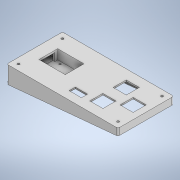
# Autodesk Inventor part: betonbase
Saved by Autodesk Inventor 2021 (Build 250183000, 183)
## iProperties
Created: 2020-07-06
Part Number: betonbase
Material: Generic
Document SubType Name: Modeling
Designer: adaml
Density: 1 g/cm^3
Appearance: Default
Author: adaml
Autodesk Inventor part; units mm, degrees
sketch "Sketch1" plane through (0, 0, 0) normal (0, 1, 0) x (-1, 0, 0)
  line L0 (-55.372, 28.575) -> (55.372, 28.575)
  line L1 (57.15, 26.797) -> (57.15, -26.797)
  line L2 (55.372, -28.575) -> (-55.372, -28.575)
  line L3 (-57.15, -26.797) -> (-57.15, 26.797)
  line L4 (-57.15, 28.575) -> (57.15, -28.575) construction
  line L5 (57.15, 28.575) -> (-57.15, -28.575) construction
  arc A0 (55.372, -28.575) -> (57.15, -26.797) centre (55.372, -26.797) ccw
  arc A1 (57.15, 26.797) -> (55.372, 28.575) centre (55.372, 26.797) ccw
  arc A2 (-57.15, -26.797) -> (-55.372, -28.575) centre (-55.372, -26.797) ccw
  arc A3 (-55.372, 28.575) -> (-57.15, 26.797) centre (-55.372, 26.797) ccw
  point P0 (0, 0)
  dimension "d0" = 114.3
  dimension "d1" = 57.15
  dimension "d2" = 1.778
  dimension "d3" = 1.778
  dimension "d4" = 1.778
  constraints: 12 end point, 8 point on circle, 8 point on line, 8 tangent, 4 centre point, 2 midpoint, 2 parallel, 1 equal radius, 1 horizontal, 1 perpendicular
  measures "d0" distance of L4.end L5.end
  measures "d1" distance of L5.start L4.end
  measures "d2" radius of A0
  measures "d3" radius of A2
  measures "d4" radius of A3
extrude "Extrusion1" add sketch "Sketch1" along normal blind 17.78
sketch "Sketch2" plane through (-55.372, 0, 28.575) normal (0, 0, 1) x (1, 0, 0)
  line L0 (112.522, 0) -> (112.522, 17.78) projected
  line L1 (112.522, 17.78) -> (112.522, 10.668)
  line L2 (0, 0) -> (-1.778, 0) projected
  line L3 (112.522, 10.668) -> (-1.778, 0)
  line L4 (-1.778, 0) -> (112.522, 0)
  line L5 (112.522, 0) -> (110.744, 0) projected
  line L6 (112.522, 10.668) -> (112.522, 0)
  point P0 (55.372, 0)
  dimension "d7" = 7.112
  constraints: 8 end point, 1 collinear, 1 point on line, 1 vertical
  measures "d7" distance of L0.end L1.end
extrude "Extrusion2" cut sketch "Sketch2" against normal blind 88.5825
sketch "Sketch4" plane through (0, 17.78, 0) normal (0, 1, 0) x (1, 0, 0)
  line L0 (-57.15, 26.797) -> (-57.15, -26.797) projected
  line L1 (-57.15, 0) -> (-51.054, 0)
  line L2 (-51.054, 0) -> (-28.702, 0)
  circle A0 centre (-28.702, 0) radius 22.352
  line L3 (-6.35, 0) -> (-1.524, 0)
  line L4 (-1.524, 0) -> (-1.524, -20.193)
  line L5 (-1.524, -20.193) -> (11.176, -20.193)
  line L6 (11.176, -20.193) -> (11.176, -13.843)
  line L7 (-1.524, -13.843) -> (11.176, -13.843)
  line L8 (11.176, -13.843) -> (11.176, 0)
  line L9 (34.544, 14.605) -> (34.544, -14.605)
  line L10 (15.494, 0) -> (34.544, 0)
  line L11 (34.544, 0) -> (15.494, 0)
  line L12 (15.494, 0) -> (15.494, 24)
  line L13 (15.494, 24) -> (34.544, 24)
  line L14 (34.544, 24) -> (34.544, 0)
  line L15 (34.544, 0) -> (15.494, 0)
  line L16 (15.494, 0) -> (15.494, -24)
  line L17 (15.494, -24) -> (34.544, -24)
  line L18 (34.544, -24) -> (34.544, 0)
  line L19 (34.544, 0) -> (53.594, 0)
  line L20 (53.594, 0) -> (53.594, -14.25)
  line L21 (53.594, -14.25) -> (34.544, -14.25)
  line L22 (34.544, -14.25) -> (34.544, 0)
  line L23 (34.544, 0) -> (53.594, 0)
  line L24 (53.594, 0) -> (53.594, 14.25)
  line L25 (53.594, 14.25) -> (34.544, 14.25)
  line L26 (34.544, 14.25) -> (34.544, 0)
  line L27 (18.019, -5) -> (32.019, -5)
  line L28 (32.019, -5) -> (32.019, -19)
  line L29 (32.019, -19) -> (18.019, -19)
  line L30 (18.019, -5) -> (32.019, -19) construction
  line L31 (32.019, -5) -> (18.019, -19) construction
  line L32 (32.019, 5) -> (18.019, 5)
  line L33 (18.019, 19) -> (32.019, 19)
  line L34 (32.019, 19) -> (32.019, 5)
  line L35 (32.019, 5) -> (18.019, 19) construction
  line L36 (18.019, 5) -> (32.019, 19) construction
  line L37 (37.069, -7) -> (51.069, -7)
  line L38 (51.069, -7) -> (51.069, 7)
  line L39 (51.069, 7) -> (37.069, 7)
  line L40 (37.069, -7) -> (51.069, 7) construction
  line L41 (51.069, -7) -> (37.069, 7) construction
  line L42 (-34.702, -6) -> (-22.702, -6)
  line L43 (-22.702, -6) -> (-22.702, 6)
  line L44 (-22.702, 6) -> (-34.702, 6)
  line L45 (-34.702, 6) -> (-34.702, -6)
  line L46 (-34.702, -6) -> (-22.702, 6) construction
  line L47 (-22.702, -6) -> (-34.702, 6) construction
  line L48 (18.269, 5.25) -> (31.769, 5.25)
  line L49 (31.769, 5.25) -> (31.769, 18.75)
  line L50 (31.769, 18.75) -> (18.269, 18.75)
  line L51 (18.269, 18.75) -> (18.269, 5.25)
  line L52 (18.269, 5.25) -> (31.769, 18.75) construction
  line L53 (31.769, 5.25) -> (18.269, 18.75) construction
  line L54 (18.269, -18.75) -> (31.769, -18.75)
  line L55 (31.769, -18.75) -> (31.769, -5.25)
  line L56 (31.769, -5.25) -> (18.269, -5.25)
  line L57 (18.269, -5.25) -> (18.269, -18.75)
  line L58 (18.269, -18.75) -> (31.769, -5.25) construction
  line L59 (31.769, -18.75) -> (18.269, -5.25) construction
  line L60 (37.319, -6.75) -> (50.819, -6.75)
  line L61 (50.819, -6.75) -> (50.819, 6.75)
  line L62 (50.819, 6.75) -> (37.319, 6.75)
  line L63 (37.319, 6.75) -> (37.319, -6.75)
  line L64 (37.319, -6.75) -> (50.819, 6.75) construction
  line L65 (50.819, -6.75) -> (37.319, 6.75) construction
  point P0 (0, 0)
  point P1 (25.019, -12)
  point P2 (25.019, 12)
  point P3 (44.069, 0)
  dimension "d15" = 6.096
  dimension "d16" = 22.352
  dimension "d17" = 4.826
  dimension "d26" = 12.7
  dimension "d52" = 19.05
  dimension "d53" = 24
  dimension "d54" = 24
  dimension "d55" = 14.25
  dimension "d56" = 14.25
  dimension "d57" = 14
  dimension "d58" = 14
  dimension "d59" = 14
  dimension "d60" = 14
  dimension "d61" = 14
  dimension "d62" = 14
  dimension "d86" = 12
  dimension "d87" = 12
  dimension "d208" = 13.5
  dimension "d209" = 13.5
  dimension "d210" = 13.5
  dimension "d211" = 13.5
  dimension "d212" = 13.5
  dimension "d213" = 13.5
  constraints: 130 end point, 19 parallel, 17 midpoint, 15 horizontal, 11 perpendicular, 2 point on circle, 2 vertical, 1 centre point, 1 coincident, 1 point on line
  measures "d15" distance of L1.start L1.end
  measures "d16" distance of L1.end L2.end
  measures "d17" distance of L3.start L3.end
  measures "d26" distance of L4.end L5.end
  measures "d52" distance of L12.end L13.end
  measures "d53" distance of L11.end L12.end
  measures "d54" distance of L16.end L15.end
  measures "d55" distance of L19.end L20.end
  measures "d56" distance of L24.end L23.end
  measures "d57" distance of L28.end L29.end
  measures "d58" distance of L27.end L28.end
  measures "d59" distance of L33.start L33.end
  measures "d60" distance of L32.end L33.start
  measures "d61" distance of L39.end L38.end
  measures "d62" distance of L38.end L37.end
  measures "d86" distance of L44.end L43.end
  measures "d87" distance of L43.end L42.end
  measures "d208" distance of L50.end L49.end
  measures "d209" distance of L49.end L48.end
  measures "d210" distance of L56.end L55.end
  measures "d211" distance of L55.end L54.end
  measures "d212" distance of L62.end L61.end
  measures "d213" distance of L61.end L60.end
shell "Shell1" thickness 2 removed faces 1 at (-18.4573, 3.6113, -9.525)
extrude "Extrusion6" cut sketch "Sketch4" against normal blind 23.8125 contours L7 L6 L5 L4 | L63 L62 L61 L19 | L19 L61 L60 L63 | L45 L44 L43 L42 | L51 L50 L49 L48 | L57 L56 L55 L54
sketch "Sketch6" plane through (-55.15, 15.78, -26.575) normal (0, -1, 0) x (1, 0, 0)
  line L0 (107.7935, 6.255) -> (70.9735, 6.255)
  line L1 (70.9735, 6.255) -> (70.9735, 46.895)
  line L2 (70.9735, 46.895) -> (107.7935, 46.895)
  line L3 (107.7935, 46.895) -> (107.7935, 6.255)
  line L4 (107.7935, 6.255) -> (70.9735, 46.895) construction
  line L5 (70.9735, 6.255) -> (107.7935, 46.895) construction
  line L6 (70.9735, 46.895) -> (51.9622, 46.895)
  line L7 (51.9622, 46.895) -> (51.9622, 6.255)
  line L8 (51.9622, 6.255) -> (70.9735, 6.255)
  line L9 (70.9735, 6.255) -> (70.9735, 46.895)
  point P0 (55.15, 26.575)
  point P1 (89.3835, 26.575)
  point P2 (70.9735, 6.255)
  dimension "d43" = 40.64
  constraints: 20 end point, 4 parallel, 2 horizontal, 2 midpoint, 2 perpendicular
  measures "d43" distance of L0.end L1.end
extrude "Extrusion7" cut sketch "Sketch6" against normal blind 0.5
ref_plane "Work Plane1" through (-57.15, 0, -26.797) normal (0.9956727, 0.0929295, 0) x (0, 0, 1)
sketch "Sketch7" plane through (-57.15, 17.78, -26.797) normal (-1, 0, 0) x (0, 0, 1)
  ellipse E0 centre (0, -17.6141) end of major axis (1.778, -17.6141) minor radius 0.1659 (-1.778, -17.6141) -> (0, -17.78) ccw projected
  line L0 (0, -17.78) -> (0, 0) projected
  line L1 (0.222, -12.7049) -> (53.372, -12.7049)
  line L2 (0, -17.78) -> (53.594, -17.78) projected
  line L3 (0.222, -12.7049) -> (0.222, -17.78)
  line L4 (26.797, -17.78) -> (26.797, -11.2738)
  line L5 (53.372, -12.7049) -> (53.372, -17.78)
  constraints: 8 end point, 2 symmetric about line, 1 perpendicular, 1 point on line, 1 vertical, 1 other
extrude "Extrusion8" cut sketch "Sketch7" against normal blind 104.775
sketch "Sketch8" plane through (-57.15, 17.78, -26.797) normal (-1, 0, 0) x (0, 0, 1)
  line L0 (0.222, -12.7049) -> (53.372, -12.7049) projected
  line L1 (6.477, -2) -> (47.117, -2) projected
  line L2 (53.372, -12.7049) -> (35.172, -12.7049)
  line L3 (44.272, -12.7049) -> (44.272, -6.5049)
  line L4 (44.272, -6.5049) -> (49.7838, -6.5049)
  line L5 (49.7838, -6.5049) -> (49.7838, -12.7049)
  line L6 (44.272, -6.5049) -> (38.7602, -6.5049)
  line L7 (38.7602, -6.5049) -> (38.7602, -12.7049)
  point P0 (26.797, -17.78)
  dimension "d91" = 18.2
  dimension "d92" = 5.5118
  dimension "d93" = 5.5118
  constraints: 12 end point, 4 point on line, 3 perpendicular, 1 midpoint, 1 vertical
  measures "d91" distance of L0.end L2.end
  measures "d92" distance of L3.end L4.end
  measures "d93" distance of L3.end L6.end
extrude "Extrusion9" cut sketch "Sketch8" against normal blind 25.4
sketch "Sketch9" plane through (-55.15, 15.78, 26.575) normal (1, 0, 0) x (0, 0, -1)
  line L0 (53.15, -10.7049) -> (0, -10.7049) projected
  line L1 (15.475, -3.5049) -> (17.475, -3.5049)
  line L2 (32.075, -4.5049) -> (32.075, -10.7049) projected
  line L3 (32.075, -7.5049) -> (32.075, -6.5049)
  line L4 (21.075, -10.7049) -> (21.075, -4.5049) projected
  line L5 (21.075, -7.5049) -> (21.075, -6.5049)
  line L6 (0, -15.78) -> (0, -5.2987) projected
  line L7 (0, -7.5049) -> (18.2, -7.5049)
  line L8 (0, -7.5049) -> (18.2, -7.5049) construction
  line L9 (18.2, -6.5049) -> (0, -6.5049)
  line L10 (18.2, -5.5049) -> (0, -5.5049)
  line L11 (14.6118, -4.5049) -> (14.6118, -10.7049) projected
  line L12 (14.6118, -8.5049) -> (14.6118, -4.5049)
  line L13 (3.5882, -10.7049) -> (3.5882, -4.5049) projected
  line L14 (3.5882, -8.5049) -> (3.5882, -4.5049)
  line L15 (18.2, -7.5049) -> (18.2, -5.5049)
  line L16 (0, -7.5049) -> (0, -5.5049)
  line L17 (18.2, -4.5049) -> (0, -4.5049)
  line L18 (18.2, -3.5049) -> (0, -3.5049)
  line L19 (18.2, -5.5049) -> (18.2, -3.5049)
  line L20 (18.2, -7.5049) -> (20.2, -7.5049)
  line L21 (20.2, -7.5049) -> (20.2, -3.5049)
  line L22 (20.2, -3.5049) -> (18.2, -3.5049)
  line L23 (0, -3.5049) -> (0, -7.5049)
  line L24 (20.2, -3.5049) -> (20.2, 0)
  line L25 (53.15, 0) -> (0, 0) projected
  line L26 (18.2, 0) -> (18.2, -3.5049)
  line L27 (20.2, 0) -> (18.2, 0)
  point P0 (26.575, -15.78)
  point P1 (3.5882, -7.5049)
  point P2 (3.5882, -6.5049)
  point P3 (14.6118, -6.5049)
  point P4 (14.6118, -7.5049)
  point P5 (17.475, -3.5049)
  point P6 (15.475, -3.5049)
  dimension "d94" = 18.2
  dimension "d95" = 0
  dimension "d96" = 2
  constraints: 42 end point, 13 point on line, 6 collinear, 3 horizontal, 3 perpendicular, 3 vertical, 2 parallel
  measures "d94" distance of L7.start L7.end
  measures "d95" distance between parallel lines of L7 L8
  measures "d96" distance of L8.end L20.end
extrude "Extrusion10" add sketch "Sketch9" along normal blind 2 contours L11 L9 L15 L7 | L6 L9 L13 L7 | L15 L19 L22 L21 L20 | L22 L26 L25 L24 | L17 L23 L18 L1 L19
ref_plane "Work Plane2" through (-21.82, 15.78, 26.575) normal (1, 0, 0) x (0, 0, -1)
sketch "Sketch10" plane through (-55.15, 15.78, -26.575) normal (0, -1, 0) x (1, 0, 0)
  line L0 (110.3, 0) -> (0, 0) projected
  line L1 (15.5947, 0) -> (15.5947, 40)
  line L2 (15.5947, 0) -> (55.5947, 0) construction
  point P0 (55.15, 26.575)
  dimension "d89" = 40
  dimension "d90" = 90
  constraints: 4 end point, 2 perpendicular, 1 horizontal, 1 point on line
  measures "d89" distance of L1.start L1.end
  measures "d90" angle of L2 L1
ref_plane "Work Plane3" through (-55.15, 9.18, -26.575) normal (0, -1, 0) x (1, 0, 0)
sketch "Sketch12" plane through (-55.15, 15.78, -26.575) normal (0, -1, 0) x (1, 0, 0)
  line L0 (32.448, 20.575) -> (32.448, 32.575) projected
  line L1 (20.448, 20.575) -> (32.448, 20.575) projected
  line L2 (32.448, 32.575) -> (20.448, 32.575)
  line L3 (20.448, 32.575) -> (20.448, 20.575)
  line L4 (20.448, 20.575) -> (32.448, 20.575)
  line L5 (32.448, 20.575) -> (32.448, 32.575)
  line L6 (32.448, 32.575) -> (32.448, 30.575)
  line L7 (32.448, 30.575) -> (36.448, 30.575)
  line L8 (36.448, 30.575) -> (36.448, 33.575)
  line L9 (36.448, 33.575) -> (32.448, 33.575)
  line L10 (32.448, 33.575) -> (32.448, 32.575)
  line L11 (20.448, 32.575) -> (20.448, 20.575) projected
  line L12 (20.448, 32.575) -> (20.448, 34.575)
  line L13 (20.448, 34.575) -> (36.448, 34.575)
  line L14 (36.448, 33.575) -> (36.448, 34.575)
  line L15 (32.448, 33.575) -> (32.448, 34.575)
  line L16 (32.448, 20.575) -> (30.948, 20.575)
  line L17 (30.948, 20.575) -> (33.948, 20.575)
  line L18 (32.448, 20.575) -> (32.448, 19.575)
  line L19 (20.448, 34.575) -> (20.448, 33.575)
  line L20 (20.448, 33.575) -> (18.448, 33.575)
  line L21 (20.448, 33.575) -> (10.448, 33.575)
  line L22 (10.448, 33.575) -> (10.448, 34.575)
  line L23 (20.448, 34.575) -> (20.448, 33.575)
  line L24 (20.448, 32.575) -> (15.448, 32.575)
  line L25 (15.448, 32.575) -> (15.448, 33.575)
  line L26 (10.448, 34.575) -> (20.448, 34.575)
  line L27 (32.448, 20.575) -> (37.448, 20.575)
  line L28 (37.448, 20.575) -> (37.448, 34.575)
  line L29 (37.448, 34.575) -> (11.448, 34.575)
  line L30 (10.448, 34.575) -> (10.448, 15.275)
  line L31 (10.448, 15.275) -> (37.448, 15.275)
  line L32 (37.448, 15.275) -> (37.448, 20.575)
  line L33 (10.448, 15.275) -> (10.448, 13.275)
  line L34 (10.448, 13.275) -> (37.448, 13.275)
  line L35 (37.448, 13.275) -> (39.448, 13.275)
  line L36 (39.448, 13.275) -> (39.448, 34.575)
  line L37 (39.448, 34.575) -> (37.448, 34.575)
  line L38 (10.448, 13.275) -> (8.448, 13.275)
  line L39 (8.448, 13.275) -> (8.448, 18.275)
  line L40 (8.448, 18.275) -> (10.448, 18.275)
  line L41 (39.448, 34.575) -> (39.448, 36.575)
  line L42 (39.448, 36.575) -> (34.448, 36.575)
  line L43 (34.448, 36.575) -> (34.448, 34.575)
  line L44 (37.448, 34.575) -> (34.448, 34.575)
  point P0 (55.15, 26.575)
  point P1 (18.448, 33.575)
  dimension "d100" = 2
  dimension "d101" = 4
  dimension "d102" = 3
  dimension "d103" = 2
  dimension "d104" = 1.5
  dimension "d105" = 3
  dimension "d106" = 1
  dimension "d107" = 1
  dimension "d108" = 2
  dimension "d109" = 10
  dimension "d113" = 5
  dimension "d114" = 5
  dimension "d115" = 14
  dimension "d116" = 26
  dimension "d117" = 19.3
  dimension "d118" = 2
  dimension "d119" = 2
  dimension "d120" = 2
  dimension "d121" = 5
  dimension "d122" = 2
  dimension "d123" = 5
  constraints: 84 end point, 19 perpendicular, 13 point on line, 4 horizontal, 4 vertical, 3 collinear, 2 midpoint, 2 parallel
  measures "d100" distance of L0.end L6.end
  measures "d101" distance of L6.end L7.end
  measures "d102" distance of L7.end L8.end
  measures "d103" distance of L12.end L2.end
  measures "d104" distance of L4.end L16.end
  measures "d105" distance of L16.end L17.end
  measures "d106" distance of L4.end L18.end
  measures "d107" distance of L12.end L19.end
  measures "d108" distance of L19.end L20.end
  measures "d109" distance of L19.end L21.end
  measures "d113" distance of L2.end L24.end
  measures "d114" distance of L0.start L27.end
  measures "d115" distance of L27.end L28.end
  measures "d116" distance of L28.end L29.end
  measures "d117" distance of L22.end L30.end
  measures "d118" distance of L30.end L33.end
  measures "d119" distance of L34.end L35.end
  measures "d120" distance of L33.end L38.end
  measures "d121" distance of L38.end L39.end
  measures "d122" distance of L36.end L41.end
  measures "d123" distance of L41.end L42.end
extrude "Extrusion12" add sketch "Sketch12" along normal blind 8 contours L28 L37 L36 L35 L34 L33 L31 L32 | L29 L13 L43 L42 L41 L37 | L33 L38 L39 L40 L30
sketch "Sketch13" plane through (-55.15, 7.78, -26.575) normal (0, -1, 0) x (1, 0, 0)
  line L0 (8.448, 18.275) -> (8.448, 13.275) projected
  line L1 (8.448, 13.275) -> (39.448, 13.275)
  line L2 (39.448, 13.275) -> (39.448, 36.575) projected
  line L3 (39.448, 13.275) -> (39.448, 36.575)
  line L4 (34.448, 36.575) -> (39.448, 36.575) projected
  line L5 (39.448, 36.575) -> (34.448, 36.575)
  line L6 (34.448, 36.575) -> (34.448, 34.575)
  line L7 (34.448, 34.575) -> (8.448, 34.575)
  line L8 (8.448, 34.575) -> (8.448, 13.275)
  point P0 (55.15, 26.575)
  point P1 (39.448, 13.275)
  constraints: 12 end point, 3 perpendicular, 2 collinear, 1 horizontal
extrude "Extrusion13" add sketch "Sketch13" along normal blind 2
sketch "Sketch14" plane through (-55.15, 15.78, -26.575) normal (0, -1, 0) x (1, 0, 0)
  line L0 (32.448, 20.575) -> (32.448, 32.575)
  line L1 (20.448, 20.575) -> (32.448, 20.575)
  line L2 (32.448, 32.575) -> (20.448, 32.575)
  line L3 (20.448, 32.575) -> (20.448, 20.575)
  line L4 (20.448, 20.575) -> (32.448, 20.575)
  line L5 (32.448, 20.575) -> (32.448, 32.575)
  line L6 (32.448, 32.575) -> (32.448, 30.575)
  line L7 (32.448, 30.575) -> (36.448, 30.575)
  line L8 (36.448, 30.575) -> (36.448, 33.575)
  line L9 (36.448, 33.575) -> (32.448, 33.575)
  line L10 (32.448, 33.575) -> (32.448, 32.575)
  line L11 (20.448, 32.575) -> (20.448, 20.575)
  line L12 (20.448, 32.575) -> (20.448, 34.575)
  line L13 (20.448, 34.575) -> (36.448, 34.575)
  line L14 (36.448, 33.575) -> (36.448, 34.575)
  line L15 (32.448, 33.575) -> (32.448, 34.575)
  line L16 (32.448, 20.575) -> (30.948, 20.575)
  line L17 (30.948, 20.575) -> (33.948, 20.575)
  line L18 (32.448, 20.575) -> (32.448, 19.575)
  line L19 (20.448, 34.575) -> (20.448, 33.575)
  line L20 (20.448, 33.575) -> (18.448, 33.575)
  line L21 (20.448, 33.575) -> (10.448, 33.575)
  line L22 (10.448, 33.575) -> (10.448, 34.575)
  line L23 (20.448, 34.575) -> (20.448, 33.575)
  line L24 (20.448, 32.575) -> (15.448, 32.575)
  line L25 (15.448, 32.575) -> (15.448, 33.575)
  line L26 (10.448, 34.575) -> (20.448, 34.575)
  line L27 (32.448, 20.575) -> (37.448, 20.575)
  line L28 (37.448, 20.575) -> (37.448, 34.575)
  line L29 (37.448, 34.575) -> (11.448, 34.575)
  line L30 (10.448, 34.575) -> (10.448, 15.275)
  line L31 (10.448, 15.275) -> (37.448, 15.275)
  line L32 (37.448, 15.275) -> (37.448, 20.575)
  line L33 (10.448, 15.275) -> (10.448, 13.275)
  line L34 (10.448, 13.275) -> (37.448, 13.275)
  line L35 (37.448, 13.275) -> (39.448, 13.275)
  line L36 (39.448, 13.275) -> (39.448, 34.575)
  line L37 (39.448, 34.575) -> (37.448, 34.575)
  line L38 (10.448, 13.275) -> (8.448, 13.275)
  line L39 (8.448, 13.275) -> (8.448, 18.275)
  line L40 (8.448, 18.275) -> (10.448, 18.275)
  line L41 (39.448, 34.575) -> (39.448, 36.575)
  line L42 (39.448, 36.575) -> (34.448, 36.575)
  line L43 (34.448, 36.575) -> (34.448, 34.575)
  line L44 (37.448, 34.575) -> (34.448, 34.575)
  point P0 (55.15, 26.575)
  point P1 (55.15, 26.575)
  point P2 (18.448, 33.575)
  point P3 (10.448, 33.575)
  dimension "d126" = 2
  dimension "d127" = 4
  dimension "d128" = 3
  dimension "d129" = 2
  dimension "d130" = 1.5
  dimension "d131" = 3
  dimension "d132" = 1
  dimension "d133" = 1
  dimension "d134" = 2
  dimension "d135" = 10
  dimension "d136" = 5
  dimension "d137" = 5
  dimension "d138" = 14
  dimension "d139" = 26
  dimension "d140" = 19.3
  dimension "d141" = 2
  dimension "d142" = 2
  dimension "d143" = 2
  dimension "d144" = 5
  dimension "d145" = 2
  dimension "d146" = 5
  constraints: 90 end point, 19 perpendicular, 13 point on line, 4 horizontal, 4 vertical, 3 collinear, 2 midpoint, 2 parallel
  measures "d126" distance of L0.end L6.end
  measures "d127" distance of L6.end L7.end
  measures "d128" distance of L7.end L8.end
  measures "d129" distance of L12.end L2.end
  measures "d130" distance of L4.end L16.end
  measures "d131" distance of L16.end L17.end
  measures "d132" distance of L4.end L18.end
  measures "d133" distance of L12.end L19.end
  measures "d134" distance of L19.end L20.end
  measures "d135" distance of L19.end L21.end
  measures "d136" distance of L2.end L24.end
  measures "d137" distance of L0.start L27.end
  measures "d138" distance of L27.end L28.end
  measures "d139" distance of L28.end L29.end
  measures "d140" distance of L22.end L30.end
  measures "d141" distance of L30.end L33.end
  measures "d142" distance of L34.end L35.end
  measures "d143" distance of L33.end L38.end
  measures "d144" distance of L38.end L39.end
  measures "d145" distance of L36.end L41.end
  measures "d146" distance of L41.end L42.end
extrude "Extrusion14" cut sketch "Sketch14" against normal blind 2 contours L17 L27 L32 L31 L30 L21 L25 L24 L3 L1 | L0 L7 L8 L14 L29 L28 L27 L17 | L0 L10 L9 L8 L7 | L2 L12 L13 L15 L10 | L24 L25 L21 L20 L12 | L15 L13 L14 L9 | L20 L21 L22 L26 L12
sketch "Sketch15" plane through (-46.702, 15.78, -13.3) normal (-1, 0, 0) x (0, 0, 1)
  line L0 (0, 0) -> (2, 0)
  line L1 (2, 0) -> (2, -10.0307)
  line L2 (2, -10.0307) -> (0, -10.0307)
  line L3 (0, -10.0307) -> (0, 0)
  line L4 (2, -10.0307) -> (21.3, -10.0307)
  line L5 (21.3, -10.0307) -> (21.3, -8.0307)
  line L6 (21.3, -8.0307) -> (2, -8.0307)
  line L7 (2, -8.0307) -> (2, -10.0307)
  point P0 (13.3, -15.78)
  point P1 (2, -8.0307)
  dimension "d149" = 2
  dimension "d150" = 2
  constraints: 16 end point, 4 parallel, 2 horizontal, 2 perpendicular
  measures "d149" distance of L1.end L2.end
  measures "d150" distance of L5.end L4.end
extrude "Extrusion15" add sketch "Sketch15" along normal blind 9.9375
sketch "Sketch16" plane through (-55.15, 8.2751, 6.375) normal (0, -1, 0) x (1, 0, 0)
  line L0 (-2, 5.5882) -> (0, 5.5882) projected
  line L1 (2, 2) -> (2, 0) projected
  line L2 (0, 5.5882) -> (2, 5.5882)
  line L3 (2, 5.5882) -> (2, 0)
  line L4 (2, 0) -> (0, 0)
  line L5 (0, 0) -> (0, 5.5882)
  point P0 (55.15, -6.375)
  constraints: 8 end point, 2 parallel, 1 horizontal, 1 perpendicular
extrude "Extrusion16" add sketch "Sketch16" along normal up to surface (3.2 mm away)
sketch "Sketch17" plane through (-55.15, 5.78, -26.575) normal (0, -1, 0) x (1, 0, 0)
  line L0 (34.448, 34.575) -> (37.448, 34.575) projected
  line L1 (34.448, 34.575) -> (37.448, 34.575)
  line L2 (37.448, 34.575) -> (37.448, 15.275) projected
  line L3 (37.448, 34.575) -> (37.448, 15.275)
  line L4 (37.448, 15.275) -> (10.448, 15.275) projected
  line L5 (37.448, 15.275) -> (10.448, 15.275)
  line L6 (10.448, 18.275) -> (10.448, 34.575) projected
  line L7 (10.448, 15.275) -> (10.448, 34.575)
  line L8 (34.448, 34.575) -> (8.448, 34.575) projected
  line L9 (10.448, 34.575) -> (34.448, 34.575)
  line L10 (10.448, 34.575) -> (10.448, 15.275) projected
  line L11 (10.448, 15.275) -> (13.948, 15.275)
  line L12 (13.948, 15.275) -> (13.948, 16.375)
  line L13 (13.948, 16.375) -> (13.948, 17.875)
  circle A0 centre (15.448, 17.875) radius 1.5
  line L14 (16.948, 17.875) -> (30.948, 17.875)
  line L15 (30.948, 17.875) -> (32.448, 17.875)
  circle A1 centre (32.448, 17.875) radius 1.5
  circle A2 centre (15.448, 17.875) radius 1
  circle A3 centre (32.448, 17.875) radius 1
  point P0 (55.15, 26.575)
  dimension "d193" = 3.5
  dimension "d194" = 1.1
  dimension "d195" = 1.5
  dimension "d196" = 14
  dimension "d197" = 1.5
  dimension "d198" = 2
  dimension "d199" = 2
  constraints: 20 end point, 4 collinear, 3 coincident, 3 point on line, 2 centre point, 2 horizontal alignment, 2 perpendicular, 1 horizontal, 4 other
  measures "d193" distance of L4.end L11.end
  measures "d194" distance of L11.end L12.end
  measures "d195" distance of L12.end L13.end
  measures "d196" distance of L14.start L14.end
  measures "d197" distance of L14.end L15.end
  measures "d198" diameter of A2
  measures "d199" diameter of A3
ref_plane "Work Plane4" through (-21.95, 11.2751, 26.575) normal (1, 0, 0) x (0, 0, -1)
sketch "Sketch18" plane through (-55.15, 15.78, -26.575) normal (0, -1, 0) x (1, 0, 0)
  line L0 (0, 53.15) -> (110.3, 53.15) projected
  line L1 (33.1965, 53.15) -> (29.1965, 53.15)
  line L2 (29.1965, 53.15) -> (33.1965, 53.15)
  line L3 (33.1965, 53.15) -> (33.1965, 49.15)
  line L4 (33.1965, 49.15) -> (35.1965, 49.15)
  line L5 (35.1965, 49.15) -> (35.1965, 53.15)
  line L6 (35.1965, 53.15) -> (33.1965, 53.15)
  line L7 (34.448, 34.575) -> (8.448, 34.575) projected
  line L8 (33.1965, 34.575) -> (37.1965, 34.575)
  line L9 (37.1965, 34.575) -> (33.1965, 34.575)
  line L10 (33.1965, 34.575) -> (33.1965, 38.575)
  line L11 (33.1965, 38.575) -> (35.1965, 38.575)
  line L12 (35.1965, 38.575) -> (35.1965, 34.575)
  line L13 (34.448, 34.575) -> (37.448, 34.575) projected
  line L14 (35.1965, 34.575) -> (35.1965, 38.575)
  point P0 (55.15, 26.575)
  dimension "d156" = 4
  dimension "d157" = 4
  dimension "d158" = 2
  dimension "d159" = 4
  dimension "d160" = 4
  constraints: 24 end point, 6 perpendicular, 5 collinear, 5 point on line
  measures "d156" distance of L1.start L1.end
  measures "d157" distance of L1.start L3.end
  measures "d158" distance of L3.end L4.end
  measures "d159" distance of L8.start L8.end
  measures "d160" distance of L8.start L10.end
extrude "Extrusion17" add sketch "Sketch18" along normal up to surface (10 mm away)
sketch "Sketch20" plane through (-55.15, 15.78, -26.575) normal (0, -1, 0) x (1, 0, 0)
  line L0 (33.1965, 38.575) -> (35.1965, 38.575) projected
  line L1 (33.1965, 34.575) -> (8.448, 34.575) projected
  line L2 (33.1965, 38.575) -> (31.1965, 38.575)
  line L3 (31.1965, 38.575) -> (31.1965, 34.575)
  line L4 (31.1965, 34.575) -> (33.1965, 34.575)
  line L5 (33.1965, 34.575) -> (33.1965, 38.575)
  line L6 (33.1965, 49.15) -> (33.1965, 53.15) projected
  line L7 (-2, 53.15) -> (110.3, 53.15) projected
  line L8 (33.1965, 49.15) -> (31.1965, 49.15)
  line L9 (31.1965, 49.15) -> (31.1965, 53.15)
  line L10 (31.1965, 53.15) -> (33.1965, 53.15)
  line L11 (33.1965, 53.15) -> (33.1965, 49.15)
  point P0 (55.15, 26.575)
  dimension "d163" = 2
  constraints: 16 end point, 4 parallel, 3 point on line, 2 horizontal, 2 perpendicular
  measures "d163" distance of L4.end L3.end
extrude "Extrusion18" add sketch "Sketch20" along normal blind 2
sketch "Sketch22" plane through (-57.15, 0, -26.797) normal (0.9956727, 0.0929295, 0) x (0, 0, 1)
  line L0 (0.222, 0) -> (0.222, -1)
  line L1 (0.222, 0) -> (0.222, -5.0532) projected
  line L2 (0.222, -1) -> (-0.778, -1)
  line L3 (-0.778, -1) -> (-0.778, -2.27)
  line L4 (53.594, 0) -> (55.372, 0) projected
  line L5 (53.594, 0) -> (53.594, -1)
  line L6 (53.594, 0) -> (53.594, -17.7031) projected
  line L7 (53.594, -1) -> (54.594, -1)
  line L8 (54.594, -1) -> (54.594, -2.27)
  line L9 (-1.778, 0) -> (-1.778, -17.5378) projected
  line L10 (-0.778, -2.27) -> (54.594, -2.27)
  line L11 (0.222, 0) -> (53.372, 0)
  line L12 (0.222, -1) -> (53.594, -1)
  line L13 (-0.778, -2.27) -> (54.594, -2.27)
  line L14 (54.594, -2.27) -> (54.594, -1)
  line L15 (54.594, -1) -> (-0.778, -1)
  line L16 (-0.778, -1) -> (-0.778, -2.27)
  point P0 (26.797, 5.3109)
  dimension "d168" = 1
  dimension "d169" = 1
  dimension "d170" = 1.27
  dimension "d171" = 1
  dimension "d172" = 1
  dimension "d173" = 1.27
  constraints: 26 end point, 5 perpendicular, 2 parallel, 2 point on line, 1 horizontal
  measures "d168" distance of L0.start L0.end
  measures "d169" distance of L0.end L2.end
  measures "d170" distance of L2.end L3.end
  measures "d171" distance of L4.start L5.end
  measures "d172" distance of L5.end L7.end
  measures "d173" distance of L7.end L8.end
extrude "Extrusion20" cut sketch "Sketch22" along normal up to surface surface through (55.15, 0, 26.797) normal (1, 0, 0)
sketch "Sketch23" plane through (-55.15, 15.78, -26.575) normal (0, -1, 0) x (1, 0, 0)
  line L0 (0, 49.5618) -> (0, 53.15) projected
  line L1 (0, 53.15) -> (0, 49.15)
  line L2 (0, 49.15) -> (4, 49.15)
  circle A0 centre (4, 49.15) radius 1.143
  line L3 (0, 0) -> (0, 13.275) projected
  line L4 (0, 0) -> (0, 4)
  line L5 (0, 0) -> (4, 0) construction
  line L6 (0, 4) -> (4, 4)
  circle A1 centre (4, 4) radius 1.143
  line L7 (-2, 0) -> (110.3, 0) projected
  line L8 (110.3, 0) -> (110.3, 4)
  line L9 (110.3, 53.15) -> (110.3, 0) projected
  line L10 (110.3, 4) -> (110.3, 0)
  line L11 (110.3, 4) -> (106.3, 4)
  circle A2 centre (106.3, 4) radius 1.143
  line L12 (110.3, 53.15) -> (110.3, 54.372) projected
  line L13 (110.3, 53.15) -> (110.3, 49.15)
  line L14 (110.3, 49.15) -> (106.3, 49.15)
  circle A3 centre (106.3, 49.15) radius 1.143
  point P0 (55.15, 26.575)
  dimension "d176" = 4
  dimension "d177" = 4
  dimension "d178" = 2.286
  dimension "d179" = 4
  dimension "d180" = 90
  dimension "d181" = 4
  dimension "d182" = 90
  dimension "d183" = 2.286
  dimension "d184" = 4
  dimension "d185" = 4
  dimension "d186" = 4
  dimension "d187" = 2.286
  dimension "d188" = 4
  dimension "d189" = 4
  dimension "d190" = 2.286
  constraints: 20 end point, 4 centre point, 4 coincident, 4 perpendicular, 3 collinear, 2 horizontal, 2 point on line
  measures "d176" distance of L0.end L1.end
  measures "d177" distance of L1.end L2.end
  measures "d178" diameter of A0
  measures "d179" distance of L3.start L4.end
  measures "d180" angle of L5 L4
  measures "d181" distance of L4.end L6.end
  measures "d182" angle of L4 L6
  measures "d183" diameter of A1
  measures "d184" distance of L7.end L8.end
  measures "d185" distance of L8.end L7.end
  measures "d186" distance of L8.end L11.end
  measures "d187" diameter of A2
  measures "d188" distance of L9.start L13.end
  measures "d189" distance of L13.end L14.end
  measures "d190" diameter of A3
extrude "Extrusion21" cut sketch "Sketch23" against normal blind 112.268
extrude "Extrusion22" cut sketch "Sketch17" against normal blind 112.268 contours A2 | A3
sketch "Sketch24" plane through (-57.15, 17.78, -26.797) normal (-1, 0, 0) x (0, 0, 1)
  line L0 (1.8673, -6.3544) -> (28.6253, -6.3544) construction
  line L1 (28.6253, -6.3544) -> (28.6253, -12.409) construction
  line L2 (28.6253, -12.409) -> (1.8673, -12.409) construction
  line L3 (1.8673, -12.409) -> (1.8673, -6.3544) construction
  line L4 (0, -15.5001) -> (0, 0) projected
  line L5 (0.222, -12.7049) -> (38.7602, -12.7049) projected
  line L6 (0, 0) -> (53.594, 0) projected
  line L7 (38.7602, -12.7049) -> (38.7602, -6.5049) projected
  line L8 (2.3434, -10.2797) -> (3.9654, -10.2797)
  spline S0 degree 2 poles (3.9654, -10.2797) (4.1535, -10.2797) (4.4557, -10.1429) (4.6723, -9.9177) (4.7892, -9.6127) (4.7892, -9.4502) knots 0 0 0 1 2 3 4 4 4
  line L9 (4.7892, -9.4502) -> (4.7892, -9.034)
  spline S1 degree 2 poles (4.7892, -9.034) (4.7892, -8.8686) (4.6581, -8.6377) (4.5013, -8.4952) (4.3673, -8.4353) (4.3673, -8.4353) knots 0 0 0 1 2 3 4 4 4
  spline S2 degree 2 poles (4.3673, -8.4353) (4.3673, -8.4353) (4.5013, -8.3869) (4.6581, -8.2643) (4.7892, -8.0391) (4.7892, -7.8624) knots 0 0 0 1 2 3 4 4 4
  line L10 (4.7892, -7.8624) -> (4.7892, -7.4262)
  spline S3 degree 2 poles (4.7892, -7.4262) (4.7892, -7.2409) (4.6581, -6.9359) (4.4357, -6.7193) (4.1336, -6.6024) (3.9654, -6.6024) knots 0 0 0 1 2 3 4 4 4
  line L11 (3.9654, -6.6024) -> (2.3434, -6.6024)
  line L12 (2.3434, -6.6024) -> (2.3434, -10.2797)
  line L13 (3.1587, -8.2301) -> (3.1587, -7.0043)
  line L14 (3.1587, -7.0043) -> (3.9768, -7.0043)
  line L15 (3.9768, -7.0043) -> (3.9768, -8.2301)
  line L16 (3.9768, -8.2301) -> (3.1587, -8.2301)
  line L17 (3.1587, -9.8692) -> (3.1587, -8.6434)
  line L18 (3.1587, -8.6434) -> (3.9768, -8.6434)
  line L19 (3.9768, -8.6434) -> (3.9768, -9.8692)
  line L20 (3.9768, -9.8692) -> (3.1587, -9.8692)
  line L21 (6.3628, -9.0539) -> (7.9848, -9.0539)
  line L22 (7.9848, -9.0539) -> (7.9848, -8.2586)
  spline S4 degree 2 poles (7.9848, -8.2586) (7.9848, -8.1018) (7.8536, -7.7997) (7.6284, -7.5631) (7.3149, -7.4205) (7.1381, -7.4205) knots 0 0 0 1 2 3 4 4 4
  line L23 (7.1381, -7.4205) -> (6.377, -7.4205)
  spline S5 degree 2 poles (6.377, -7.4205) (6.2117, -7.4205) (5.9124, -7.5631) (5.6815, -7.7997) (5.5475, -8.1018) (5.5475, -8.2586) knots 0 0 0 1 2 3 4 4 4
  line L24 (5.5475, -8.2586) -> (5.5475, -9.4359)
  spline S6 degree 2 poles (5.5475, -9.4359) (5.5475, -9.587) (5.6815, -9.892) (5.9067, -10.1315) (6.206, -10.2797) (6.377, -10.2797) knots 0 0 0 1 2 3 4 4 4
  line L25 (6.377, -10.2797) -> (7.1381, -10.2797)
  spline S7 degree 2 poles (7.1381, -10.2797) (7.2949, -10.2797) (7.5971, -10.1486) (7.8394, -9.9177) (7.9848, -9.6241) (7.9848, -9.4616) knots 0 0 0 1 2 3 4 4 4
  line L26 (7.9848, -9.4616) -> (7.5828, -9.4616)
  spline S8 degree 2 poles (7.5828, -9.4616) (7.5828, -9.5499) (7.5058, -9.6953) (7.3776, -9.8036) (7.2122, -9.8692) (7.1239, -9.8692) knots 0 0 0 1 2 3 4 4 4
  line L27 (7.1239, -9.8692) -> (6.3628, -9.8692)
  line L28 (6.3628, -9.8692) -> (6.3628, -9.0539)
  line L29 (7.1666, -8.6463) -> (6.3628, -8.6463)
  line L30 (6.3628, -8.6463) -> (6.3628, -7.8225)
  line L31 (6.3628, -7.8225) -> (7.1666, -7.8225)
  line L32 (7.1666, -7.8225) -> (7.1666, -8.6463)
  line L33 (7.5486, -6.3572) -> (7.141, -6.3572)
  line L34 (7.141, -6.3572) -> (6.4511, -7.1754)
  line L35 (6.4511, -7.1754) -> (6.8588, -7.1754)
  line L36 (6.8588, -7.1754) -> (7.5486, -6.3572)
  line L37 (9.202, -6.6024) -> (9.202, -7.4205)
  line L38 (9.202, -7.4205) -> (8.8086, -7.4205)
  line L39 (8.8086, -7.4205) -> (8.8086, -7.8282)
  line L40 (8.8086, -7.8282) -> (9.202, -7.8282)
  line L41 (9.202, -7.8282) -> (9.202, -9.8293)
  spline S9 degree 2 poles (9.202, -9.8293) (9.202, -9.9177) (9.2761, -10.0773) (9.3987, -10.2056) (9.5668, -10.2797) (9.6552, -10.2797) knots 0 0 0 1 2 3 4 4 4
  line L42 (9.6552, -10.2797) -> (10.4249, -10.2797)
  line L43 (10.4249, -10.2797) -> (10.4249, -9.8692)
  line L44 (10.4249, -9.8692) -> (10.0172, -9.8692)
  line L45 (10.0172, -9.8692) -> (10.0172, -7.8282)
  line L46 (10.0172, -7.8282) -> (10.4249, -7.8282)
  line L47 (10.4249, -7.8282) -> (10.4249, -7.4205)
  line L48 (10.4249, -7.4205) -> (10.0172, -7.4205)
  line L49 (10.0172, -7.4205) -> (10.0172, -6.6024)
  line L50 (10.0172, -6.6024) -> (9.202, -6.6024)
  line L51 (12.0782, -10.2797) -> (12.8536, -10.2797)
  spline S10 degree 2 poles (12.8536, -10.2797) (13.0418, -10.2797) (13.3496, -10.1457) (13.5691, -9.9205) (13.6917, -9.6127) (13.6917, -9.4359) knots 0 0 0 1 2 3 4 4 4
  line L52 (13.6917, -9.4359) -> (13.6917, -8.2586)
  spline S11 degree 2 poles (13.6917, -8.2586) (13.6917, -8.0933) (13.5691, -7.7883) (13.3496, -7.5574) (13.0418, -7.4205) (12.8536, -7.4205) knots 0 0 0 1 2 3 4 4 4
  line L53 (12.8536, -7.4205) -> (12.0782, -7.4205)
  spline S12 degree 2 poles (12.0782, -7.4205) (11.9015, -7.4205) (11.5993, -7.5574) (11.3741, -7.7883) (11.2459, -8.0933) (11.2459, -8.2586) knots 0 0 0 1 2 3 4 4 4
  line L54 (11.2459, -8.2586) -> (11.2459, -9.4359)
  spline S13 degree 2 poles (11.2459, -9.4359) (11.2459, -9.6127) (11.3684, -9.9205) (11.5879, -10.1457) (11.893, -10.2797) (12.0782, -10.2797) knots 0 0 0 1 2 3 4 4 4
  line L55 (12.8793, -9.8692) -> (12.0611, -9.8692)
  line L56 (12.0611, -9.8692) -> (12.0611, -7.8282)
  line L57 (12.0611, -7.8282) -> (12.8793, -7.8282)
  line L58 (12.8793, -7.8282) -> (12.8793, -9.8692)
  line L59 (16.1147, -7.4205) -> (14.5155, -7.4205)
  line L60 (14.5155, -7.4205) -> (14.5155, -10.2797)
  line L61 (14.5155, -10.2797) -> (15.3308, -10.2797)
  line L62 (15.3308, -10.2797) -> (15.3308, -7.8282)
  line L63 (15.3308, -7.8282) -> (16.1489, -7.8282)
  line L64 (16.1489, -7.8282) -> (16.1489, -10.2797)
  line L65 (16.1489, -10.2797) -> (16.9642, -10.2797)
  line L66 (16.9642, -10.2797) -> (16.9642, -8.2586)
  spline S14 degree 2 poles (16.9642, -8.2586) (16.9642, -8.1018) (16.8302, -7.7968) (16.5993, -7.5631) (16.2915, -7.4205) (16.1147, -7.4205) knots 0 0 0 1 2 3 4 4 4
  line L67 (19.2704, -7.01) -> (18.2413, -7.8424)
  line L68 (18.2413, -7.8424) -> (18.2413, -8.2358)
  line L69 (18.2413, -8.2358) -> (19.4129, -8.2358)
  line L70 (19.4129, -8.2358) -> (19.4129, -9.8721)
  line L71 (19.4129, -9.8721) -> (18.609, -9.8721)
  spline S15 degree 2 poles (18.609, -9.8721) (18.4123, -9.8721) (18.1729, -9.6355) (18.1729, -9.4502) knots 0 0 0 1 2 2 2
  line L72 (18.1729, -9.4502) -> (17.7652, -9.4502)
  spline S16 degree 2 poles (17.7652, -9.4502) (17.7652, -9.607) (17.9078, -9.9063) (18.1444, -10.1372) (18.4465, -10.2797) (18.609, -10.2797) knots 0 0 0 1 2 3 4 4 4
  line L73 (18.609, -10.2797) -> (19.3986, -10.2797)
  spline S17 degree 2 poles (19.3986, -10.2797) (19.5554, -10.2797) (19.8547, -10.1372) (20.0856, -9.9063) (20.2282, -9.607) (20.2282, -9.4502) knots 0 0 0 1 2 3 4 4 4
  line L74 (20.2282, -9.4502) -> (20.2282, -8.6064)
  spline S18 degree 2 poles (20.2282, -8.6064) (20.2282, -8.4496) (20.0856, -8.1702) (19.8547, -7.9536) (19.5554, -7.831) (19.3986, -7.831) knots 0 0 0 1 2 3 4 4 4
  line L75 (19.3986, -7.831) -> (19.162, -7.831)
  line L76 (19.162, -7.831) -> (20.2282, -7.01)
  line L77 (20.2282, -7.01) -> (20.2282, -6.6053)
  line L78 (20.2282, -6.6053) -> (17.7852, -6.6053)
  line L79 (17.7852, -6.6053) -> (17.7852, -7.01)
  line L80 (17.7852, -7.01) -> (19.2704, -7.01)
  point P0 (26.797, -17.78)
  dimension "d202" = 1.8673
  dimension "d204" = 6.3544
  dimension "d205" = 10.1349
  constraints: 2 other
  measures "d202" distance between parallel lines of L4 L3
  measures "d204" distance between parallel lines of L6 L0
  measures "d205" distance between parallel lines of L7 L1
emboss "Emboss1" sketch "Sketch24" operation add depth 0.5 direction (1, 0, 0)
body "Solid1"
